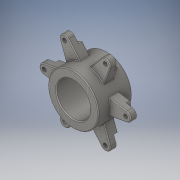
# Autodesk Inventor part: carrier
Saved by Autodesk Inventor 2018 (Build 220112000, 112)
## iProperties
Created: 2018-06-30
Part Number: carrier
Material: Stainless Steel
Document SubType Name: Modeling
Designer: Owner
Density: 8 g/cm^3
Appearance: Satin Brushed
Mass: 663.145 g
Surface Area: 220.727 cm^2
Volume: 82.8932 cm^3
Author: Owner
Autodesk Inventor part; units mm, degrees
ref_plane "YZ Plane" through (0, 0, 0) normal (1, 0, 0) x (0, 1, 0)
sketch "Sketch2" plane through (0, 0, 0) normal (0, 0, 1) x (1, 0, 0)
  circle A0 centre (0, 0) radius 20
  circle A1 centre (0, 0) radius 30
  dimension "innerdia" = 40
  dimension "Outerdia" = 60
  constraints: 2 centre point, 2 coincident
  measures "innerdia" diameter of A0
  measures "Outerdia" diameter of A1
extrude "Extrusion1" add sketch "Sketch2" along normal mid plane 40
ref_plane "Work Plane1" through (0, 0, 0) normal (0, 0, -1) x (-1, 0, 0)
sketch "Sketch4" plane through (0, 0, 0) normal (0, 0, -1) x (-1, 0, 0)
  line L0 (28.4166, 9.6175) -> (49.4496, 5.9088)
  arc A0 (49.4496, -5.9088) -> (49.4496, 5.9088) centre (48.4077, 0) ccw
  line L1 (49.4496, -5.9088) -> (28.4166, -9.6175)
  circle A1 centre (0, 0) radius 30 projected
  line L2 (0, 0) -> (46.6159, 0) construction
  dimension "Rad" = 6
  dimension "Degree" = 20
  constraints: 6 end point, 4 point on circle, 2 tangent, 1 centre point, 1 horizontal, 1 point on line, 1 other
  measures "Rad" radius of A0
  measures "Degree" angle of L1 L0
extrude "Extrusion2" add sketch "Sketch4" along normal mid plane 12 contours L0 A0 L1 A1
pattern_circular "Circular Pattern1" count 6 over 360 about axis through (0, 0, 0) along (0, 0, 1) of "Extrusion2"
fillet "Fillet1" radius 1 26 edges at (28.4166, -9.6175, 0) (29.6015, -4.8735, -6) (29.6015, 4.8735, -6) (29.6015, 4.8735, 6) (28.4166, 9.6175, 0) (29.6015, -4.8735, 6) (15, 25.9808, 6) (5.8793, 29.4183, 0) (15, 25.9808, -6) (22.5373, 19.8007, 0) (-15, 25.9808, 6) (-22.5373, 19.8007, 0) (-15, 25.9808, -6) (-5.8793, 29.4183, 0) (-28.4166, 9.6175, 0) (-30, 0, -6) (-30, 0, 6) (-28.4166, -9.6175, 0) (-15, -25.9808, 6) (-5.8793, -29.4183, 0) (-15, -25.9808, -6) (-22.5373, -19.8007, 0) (15, -25.9808, 6) (22.5373, -19.8007, 0) (15, -25.9808, -6) (5.8793, -29.4183, 0)
fillet "Fillet1" radius 1 40 edges at (38.9331, -7.7632, -6) (38.9331, -7.7632, 6) (54.4077, 0, -6) (54.4077, 0, 6) (38.9331, 7.7632, -6) (-30, 0, -20) (-30, 0, 20) (38.9331, 7.7632, 6) (-20, 0, -20) (-20, 0, 20) (26.1897, 29.8355, 6) (27.2038, 47.1184, 6) (12.7434, 37.5986, 6) (12.7434, 37.5986, -6) (26.1897, 29.8355, -6) (27.2038, 47.1184, -6) (-12.7434, 37.5986, 6) (-27.2038, 47.1184, 6) (-26.1897, 29.8355, 6) (-26.1897, 29.8355, -6) (-12.7434, 37.5986, -6) (-27.2038, 47.1184, -6) (-38.9331, 7.7632, -6) (-38.9331, 7.7632, 6) (-54.4077, 0, -6) (-38.9331, -7.7632, -6) (-54.4077, 0, 6) (-38.9331, -7.7632, 6) (-26.1897, -29.8355, 6) (-27.2038, -47.1184, 6) (-12.7434, -37.5986, 6) (-12.7434, -37.5986, -6) (-26.1897, -29.8355, -6) (-27.2038, -47.1184, -6) (12.7434, -37.5986, 6) (27.2038, -47.1184, 6) (26.1897, -29.8355, 6) (26.1897, -29.8355, -6) (12.7434, -37.5986, -6) (27.2038, -47.1184, -6)
hole "Hole1" at (48.4077, 0, 6) direction (0, 0, -1) diameter 4.917 end through all thread size "M6x1" class "6H" standard "ISO Metric profile"
pattern_circular "Circular Pattern2" count 6 over 360 about axis through (0, 0, 0) along (0, 0, 1) of "Hole1"
ref_plane "Work Plane2" through (41.4802, -71.8457, 5) normal (0.8660254, 0.5, 0) x (0, 0, 1)
sketch "Sketch5" plane through (41.4802, -71.8457, 5) normal (0.8660254, 0.5, 0) x (0, 0, 1)
  line L0 (0, -28.5526) -> (-10, -28.5526) projected
  line L1 (-11, -33.6844) -> (-11, -53.1056) projected
  line L2 (-6, -28.5526) -> (-11, -28.5526)
  line L3 (-11, -28.5526) -> (-11, -40.5526)
  line L4 (-11, -40.5526) -> (-6, -40.5526)
  line L5 (-6, -40.5526) -> (-6, -28.5526)
  line L6 (-33, -82.9603) -> (23, -82.9603) projected
  point P0 (-5, -82.9603)
  dimension "d34" = 12
  dimension "d35" = 5
  constraints: 8 end point, 2 parallel, 2 point on line, 1 horizontal, 1 perpendicular
  measures "d34" distance of L4.end L2.start
  measures "d35" distance of L3.end L4.end
revolve "Revolution1" cut sketch "Sketch5" angle 360 about axis through (0, 0, -10) along (0, 0, 1)
body "Solid1"
